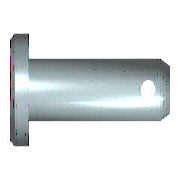
# Autodesk Inventor part: DS51F1496-07
Saved by Autodesk Inventor 2011 (Build 150239000, 239)
## iProperties
IsCustomPart: 1
Manager: MANNY MANAGER
Company: ACME
Category: DATASETS
Created: 2009-11-19
Part Number: DS51F1496-07
Material: Steel, Mild
Description: CLEVIS PINS AND COTTER PINS - CLEVIS PIN
Document SubType Name: Modeling
Standard: ANSI B18.8.1
Designer: JOE DESIGNER
Standard Revision: 1994
Standards Organization: ANSI
Language: en-US
Size Designation: PIN. CLEVIS. 0.1875 x 0.58
Categories: <MemberInstance><Categories><Category DisplayName="Fasteners" InternalName="e4da775c-781d-43d5-af7c-5136215cf5a6" Mnemonic="FSTN"><Category DisplayName="Pins" InternalName="3b3d1810-ac9b-4ede-8c7f-cc6b956350b0" Mnemonic="PIN"><CategoryParameter DisplayName="Nominal Diameter" InternalName="6cc331d7-8ea1-4fca-9c9a-55ec966217e5" Mnemonic="nomdia"/><CategoryParameter DisplayName="Nominal Length" InternalName="897bd938-6adf-4e3c-a2d4-0d7cae45eecd" Mnemonic="nomlen"/><Category DisplayName="Clevis Pins" InternalName="4b089753-0276-4279-8372-6376cec148ca" Mnemonic="CLVPIN"><CategoryParameter DisplayName="Functional Length" InternalName="559ecc49-03ee-43cf-bf76-5b0abe06f3ba" Mnemonic="fnclen"/><Category DisplayName="Clevis Pins With Head" InternalName="462db250-c675-45ed-aefa-a0efc4518892" Mnemonic="CLVPINSH"><CategoryParameter DisplayName="Head Diameter" InternalName="31cf2fff-8354-4e55-86cb-90faf880c8c9" Mnemonic="headdia"/><CategoryParameter DisplayName="Head Height" InternalName="45d740ed-44eb-4568-a895-0f0486773718" Mnemonic="headh"/><Category DisplayName="Drilled Shank" InternalName="e8552798-4a93-481f-8f00-846ab6c4d44e" Mnemonic="CLVPINSHDS"><CategoryParameter DisplayName="Hole diameter for Split Pin" InternalName="ceed0519-20f2-44b6-9878-24cf728bbc99" Mnemonic="SplitHoleDia"/><CategoryParameter DisplayName="Hole distance" InternalName="9f0dacbf-c792-4ef9-9fd6-14e6291d80cd" Mnemonic="HoleDist"/></Category></Category></Category></Category></Category><Category DisplayName="DataType" InternalName="23b78d0f-2648-40c6-8793-ca6db495c9e8" Mnemonic="DATATYPE"><CategoryParameter DisplayName="DisplayName" InternalName="05415f3d-3907-474b-a020-eb9d644f4cf3" Mnemonic="DISPLAYNAME"/><CategoryParameter DisplayName="InternalName" InternalName="cf1d0246-76d9-4b4a-8305-fa0409afb5c1" Mnemonic="INTERNALNAME"/><CategoryParameter DisplayName="Folder Name" InternalName="3f06958e-8713-4116-9be7-ed6184ecc97b" Mnemonic="FOLDERNAME"/><CategoryParameter DisplayName="Family Version" InternalName="914462f6-6e19-4b14-ba84-155b9680b1d0" Mnemonic="FAMILYREVISION"/><CategoryParameter DisplayName="ClipFormat" InternalName="bc51e27b-3422-4e78-93ef-cec197ddf230" Mnemonic="CLIPFORMAT"/><CategoryParameter DisplayName="IsMetric" InternalName="e2385c5b-1ea4-4823-96a8-8de651266ec3" Mnemonic="ISMETRIC"/><CategoryParameter DisplayName="Description" InternalName="13903e3d-64b1-4950-80da-f627842ea37f" Mnemonic="DESCRIPTION"/><CategoryParameter DisplayName="StdsOrg" InternalName="8f5914e1-4693-403f-8ab5-d37768198c9d" Mnemonic="STDSORG"/><CategoryParameter DisplayName="Standard" InternalName="0c0a119c-1e12-4c84-803f-101930972f5e" Mnemonic="STANDARD"/><CategoryParameter DisplayName="Manufacturer" InternalName="cd6c7a72-a28a-4e50-99a9-2c7f4e13e5ad" Mnemonic="MANUFACTURER"/><CategoryParameter DisplayName="Member Revision" InternalName="a65d44b9-392f-4f4f-857b-e4b3d54996fe" Mnemonic="MEMBERREVISION"/><CategoryParameter DisplayName="Standard Revision" InternalName="91d5a463-65c2-4fde-b823-3b7fea5e8e17" Mnemonic="STANDARDREVISION"/><CategoryParameter DisplayName="Revision Guid" InternalName="45a75005-10b1-4dfc-8d6d-dfe629f0b93c" Mnemonic="REVISIONGUID"/><CategoryParameter DisplayName="Designation" InternalName="2675968c-4ce5-49e0-a4f5-552d29089031" Mnemonic="DESIGNATION"/><CategoryParameter DisplayName="FileName" InternalName="8b46a4cc-9585-4fed-90c3-899f57e09a73" Mnemonic="FILENAME"/><CategoryParameter DisplayName="Default Row" InternalName="2af9ec52-faaa-4026-b378-f9fa4afca842" Mnemonic="DEFAULTROW"/><Category DisplayName="Part" InternalName="c0e0b642-3bcb-4cc8-9e80-f96d35c4afa4" Mnemonic="PART"><CategoryParameter DisplayName="Material" InternalName="818a152a-d3c3-49ca-80ee-df7d91421b8e" Mnemonic="MATERIAL"/><CategoryParameter DisplayName="Material Key" InternalName="5c9a8adb-dd2b-4535-b97f-0a94a95fe41f" Mnemonic="MATERIALKEY"/><CategoryParameter DisplayName="Part Number" InternalName="016b6077-bfbe-49bd-92c9-d8d59c39c941" Mnemonic="PARTNUMBER"/><CategoryParameter DisplayName="Stock Number" InternalName="4dba7c1c-e26c-444e-836c-b08b433409a8" Mnemonic="STOCKNUMBER"/></Category></Category><Category DisplayName="Legacy Map DA" InternalName="924fff40-ddd0-4eff-ad42-30e3774ef79e" Mnemonic="LEGACYMAPDA"><CategoryParameter DisplayName="DACookie" InternalName="316934ee-8fe1-4c7a-9c36-f2d79e1add1a" Mnemonic="DACOOKIE"/></Category><Category DisplayName="LegacyMap" InternalName="cd87c42b-3e48-431e-b5c0-1cbeb14dfe77" Mnemonic="LEGACYMAP"><CategoryParameter DisplayName="CatalogName" InternalName="d99d1e27-aa94-4de2-af4c-c348882a6f4f" Mnemonic="CATALOGNAME"/><CategoryParameter DisplayName="FamilyNumber" InternalName="e705e1f4-09cb-413e-91f9-551b4188271e" Mnemonic="FAMILYNUMBER"/><CategoryParameter DisplayName="MemberID" InternalName="8e5e0294-fc51-4c8f-b3d7-003dc5ed94f6" Mnemonic="MEMBERID"/><CategoryParameter DisplayName="unique CC member ID" InternalName="5193edd4-b2b0-4ab4-9d54-de900eee34e0" Mnemonic="CCCOOKIE"/><CategoryParameter DisplayName="unique DA member ID" InternalName="0918ad47-427f-4fed-ae26-24c81c58f590" Mnemonic="DACOOKIE"/><CategoryParameter DisplayName="Merge11 ID" InternalName="0ee8fb18-e2ed-4f39-96f6-1f4b5f50aa71" Mnemonic="MERGE11"/><CategoryParameter DisplayName="Split ID" InternalName="72b5c83c-be7f-45c4-ae51-9160ea6deb26" Mnemonic="SPLIT"/></Category></Categories><FamilyTemplate Id="si0166"><FamilyTemplateParameters><FamilyTemplateParameter ObjectType="kUserParameterObject" ValueType="xs:double" Id="1" ObjectReferenceKey="NLG"/><FamilyTemplateParameter ObjectType="kUserParameterObject" ValueType="xs:double" Id="2" ObjectReferenceKey="FAWI1"/><FamilyTemplateParameter ObjectType="kUserParameterObject" ValueType="xs:double" Id="3" ObjectReferenceKey="KOD"/><FamilyTemplateParameter ObjectType="kUserParameterObject" ValueType="xs:double" Id="4" ObjectReferenceKey="BOR"/><FamilyTemplateParameter ObjectType="kUserParameterObject" ValueType="xs:double" Id="5" ObjectReferenceKey="DIST"/><FamilyTemplateParameter ObjectType="kUserParameterObject" ValueType="xs:double" Id="6" ObjectReferenceKey="PHH2"/><FamilyTemplateParameter ObjectType="kUserParameterObject" ValueType="xs:double" Id="7" ObjectReferenceKey="PHH1"/><FamilyTemplateParameter ObjectType="kUserParameterObject" ValueType="xs:double" Id="8" ObjectReferenceKey="FAWI2"/><FamilyTemplateParameter ObjectType="kUserParameterObject" ValueType="xs:double" Id="9" ObjectReferenceKey="KOH"/><FamilyTemplateParameter ObjectType="kUserParameterObject" ValueType="xs:double" Id="10" ObjectReferenceKey="NND"/><FamilyTemplateParameter ObjectType="kPropertyObject" ValueType="xs:string" Id="100" ObjectReferenceKey="{32853F0F-3444-11d1-9E93-0060B03C1CA6}" SubObjectId="52"/><FamilyTemplateParameter ObjectType="kPropertyObject" ValueType="xs:string" Id="105" ObjectReferenceKey="{32853F0F-3444-11d1-9E93-0060B03C1CA6}" SubObjectId="5"/><FamilyTemplateParameter ObjectType="kPartComponentDefinitionObject" ValueType="xs:string" Id="110" SubObjectId="Material"/></FamilyTemplateParameters></FamilyTemplate><CategoryParameterMap><ParamToTemplateMap><ParamToTemplate CategoryParameter="//CategoryParameter[@InternalName='05415f3d-3907-474b-a020-eb9d644f4cf3']" ConstantValue="ANSI/ASME B18.8.1"/><ParamToTemplate CategoryParameter="//CategoryParameter[@InternalName='cf1d0246-76d9-4b4a-8305-fa0409afb5c1']" ConstantValue="6ae5f7ed-b510-42b6-94d6-a16557dad5f7"/><ParamToTemplate CategoryParameter="//CategoryParameter[@InternalName='3f06958e-8713-4116-9be7-ed6184ecc97b']" ConstantValue="ANSI ASME B18.8.1(1)"/><ParamToTemplate CategoryParameter="//CategoryParameter[@InternalName='914462f6-6e19-4b14-ba84-155b9680b1d0']" ConstantValue="10"/><ParamToTemplate CategoryParameter="//CategoryParameter[@InternalName='bc51e27b-3422-4e78-93ef-cec197ddf230']" ConstantValue="CF_INVENTOR.STDPARTS"/><ParamToTemplate CategoryParameter="//CategoryParameter[@InternalName='e2385c5b-1ea4-4823-96a8-8de651266ec3']" ConstantValue="false"/><ParamToTemplate CategoryParameter="//CategoryParameter[@InternalName='13903e3d-64b1-4950-80da-f627842ea37f']" ConstantValue="Clevis Pins and Cotter Pins - Clevis Pin"/><ParamToTemplate CategoryParameter="//CategoryParameter[@InternalName='8f5914e1-4693-403f-8ab5-d37768198c9d']" ConstantValue="ANSI"/><ParamToTemplate CategoryParameter="//CategoryParameter[@InternalName='0c0a119c-1e12-4c84-803f-101930972f5e']" ConstantValue="ANSI B18.8.1"/><ParamToTemplate CategoryParameter="//CategoryParameter[@InternalName='cd6c7a72-a28a-4e50-99a9-2c7f4e13e5ad']" TemplateParameter="104"/><ParamToTemplate CategoryParameter="//CategoryParameter[@InternalName='91d5a463-65c2-4fde-b823-3b7fea5e8e17']" ConstantValue="1994"/><ParamToTemplate CategoryParameter="//CategoryParameter[@InternalName='45a75005-10b1-4dfc-8d6d-dfe629f0b93c']" ConstantValue="fa0597d6-b076-4735-a8ee-70f8495f6023"/><ParamToTemplate CategoryParameter="//CategoryParameter[@InternalName='2af9ec52-faaa-4026-b378-f9fa4afca842']" ConstantValue="1"/><ParamToTemplate CategoryParameter="//CategoryParameter[@InternalName='d99d1e27-aa94-4de2-af4c-c348882a6f4f']" ConstantValue="ANSI"/><ParamToTemplate CategoryParameter="//CategoryParameter[@InternalName='e705e1f4-09cb-413e-91f9-551b4188271e']" ConstantValue="1179"/><ParamToTemplate CategoryParameter="//CategoryParameter[@InternalName='8b46a4cc-9585-4fed-90c3-899f57e09a73']" ConstantValue="ANSI B18.8.1 - PIN. CLEVIS. 0.1875 x 0.58"/><ParamToTemplate CategoryParameter="//CategoryParameter[@InternalName='a65d44b9-392f-4f4f-857b-e4b3d54996fe']" ConstantValue="a24e5c83-c57f-4104-b05d-c01beab01b9e"/><ParamToTemplate CategoryParameter="//CategoryParameter[@InternalName='6cc331d7-8ea1-4fca-9c9a-55ec966217e5']" ConstantValue="0.1875"/><ParamToTemplate CategoryParameter="//CategoryParameter[@InternalName='559ecc49-03ee-43cf-bf76-5b0abe06f3ba']" ConstantValue="0.4535"/><ParamToTemplate CategoryParameter="//CategoryParameter[@InternalName='8e5e0294-fc51-4c8f-b3d7-003dc5ed94f6']" ConstantValue="1"/><ParamToTemplate CategoryParameter="//CategoryParameter[@InternalName='316934ee-8fe1-4c7a-9c36-f2d79e1add1a']" ConstantValue="*Ans~A1881~3/16 x 0.5800~0.58*"/><ParamToTemplate CategoryParameter="//CategoryParameter[@InternalName='ceed0519-20f2-44b6-9878-24cf728bbc99']" TemplateParameter="4"/><ParamToTemplate CategoryParameter="//CategoryParameter[@InternalName='2675968c-4ce5-49e0-a4f5-552d29089031']" TemplateParameter="100"/><ParamToTemplate CategoryParameter="//CategoryParameter[@InternalName='9f0dacbf-c792-4ef9-9fd6-14e6291d80cd']" TemplateParameter="5"/><ParamToTemplate CategoryParameter="//CategoryParameter[@InternalName='31cf2fff-8354-4e55-86cb-90faf880c8c9']" TemplateParameter="3"/><ParamToTemplate CategoryParameter="//CategoryParameter[@InternalName='45d740ed-44eb-4568-a895-0f0486773718']" TemplateParameter="9"/><ParamToTemplate CategoryParameter="//CategoryParameter[@InternalName='818a152a-d3c3-49ca-80ee-df7d91421b8e']" TemplateParameter="110"/><ParamToTemplate CategoryParameter="//CategoryParameter[@InternalName='897bd938-6adf-4e3c-a2d4-0d7cae45eecd']" TemplateParameter="1"/><ParamToTemplate CategoryParameter="//CategoryParameter[@InternalName='016b6077-bfbe-49bd-92c9-d8d59c39c941']" TemplateParameter="105"/></ParamToTemplateMap></CategoryParameterMap></MemberInstance>
Density: 7.86 g/cm^3
Project: IV2010 TO 2011 UPDATE
Checked By: CHUCK CHECKER
Engr Approved By: ED ENGINEER
Mfg Approved By: DUNN RITE
Engineer: ERNIE ENGINEER
Stock Number: F1496
Mass: 1.68786 g
Surface Area: 2.63211 cm^2
Volume: 0.214741 cm^3
Author: Joe Designer
Title: STILLSON WRENCH
Subject: Simplification for Simulation
Revision Number: 0
Comments: To use for Exercise: Rules Using Spreadsheets, Forms, and Triggers
Autodesk Inventor part; units mm, degrees
ref_plane "YZ Plane" through (0, 0, 0) normal (1, 0, 0) x (0, 1, 0)
ref_plane "XZ Plane" through (0, 0, 0) normal (0, 1, 0) x (-1, 0, 0)
sketch "Sketch1" plane through (0, 0, 0) normal (0, 0, 1) x (1, 0, 0)
  line L0 (-1.8, 0) -> (-1.8, 3.5)
  line L1 (-1.8, 3.5) -> (0, 3.5)
  line L2 (0, 3.5) -> (0, 2)
  line L3 (0, 2) -> (12.5, 2)
  line L4 (12.5, 2) -> (12.5, 0)
  line L5 (-1.8, 0) -> (12.5, 0)
  line L6 (-4.7305, 0) -> (15.7829, 0) projected
  line L7 (0, -1.84) -> (0, 4.39) projected
  circle A0 centre (10.25, 0) radius 0.95
  dimension "d0" = 4
  dimension "d1" = 7
  dimension "d2" = 1.8
  dimension "d3" = 12.5
  dimension "d5" = 2.25
  dimension "d6" = 1.9
  constraints: 12 end point, 3 parallel, 2 collinear, 2 perpendicular, 1 centre point, 1 point on line, 1 vertical
  measures "d0" diameter of L3 L5
  measures "d1" diameter of L1 L5
  measures "d2" distance of L0.end L1.end
  measures "d3" distance of L2.end L3.end
  measures "d5" distance from line of L4 A0.centre
  measures "d6" diameter of A0
revolve "Body" add sketch "Sketch1" angle 360 about axis through (-1.8, 0, 0) along (1, 0, 0) picked at (10.3623, 0.2961) contours L0 L1 L2 L7 L5 | L7 L3 L4 L5 A0 | A0 L5
extrude "Hole" [suppressed]
chamfer "Chamfer1" distance 0.5 angle 45 1 edges at (-1.8, -3.5, 0) measured on face at (-1.2, 3.4547, -0.5614)
chamfer "Chamfer2" distance 0.9 angle 20 1 edges at (12.5, -2, 0) measured on face at (4.1667, 1.9935, -0.1609)
ref_plane "Work Plane1" through (6.25, 0, 2) normal (0, 0, 1) x (1, 0, 0)
equation "\"d0\" = NND"
equation "\"d1\" = KOD"
equation "\"d2\" = KOH"
equation "\"d3\" = NLG"
equation "\"d5\" = DIST"
equation "\"d6\" = BOR"
equation "\"d7\" = NND"
equation "\"d9\" = PHH2"
equation "\"d10\" = FAWI2"
equation "\"d16\" = PHH2"
equation "\"d11\" = PHH1"
equation "\"d12\" = FAWI1"
equation "\"d17\" = PHH1"
equation "\"PHH1\" = 0.9"
equation "\"PHH2\" = 0.5"
equation "\"KOD\" = 7"
equation "\"KOH\" = 1.8"
equation "\"NND\" = 4"
equation "\"FAWI1\" = 20deg"
equation "\"FAWI2\" = 45deg"
equation "\"DIST\" = 2.25"
equation "\"BOR\" = 1.9"
equation "\"NLG\" = 12.5"
body "Solid1"
